Autodesk Fusion 360 part; units mm, degrees
(part 2 of 2)
sketch "Skizze6" plane through (0, 45, 0) normal (0, 1, 0) x (-1, 0, 0) in component "Board"
  circle A0 centre (45, 23.5) radius 1.5
  circle A1 centre (-94.5, -90.5) radius 1.5
  circle A2 centre (45, -90.5) radius 1.5
  circle A3 centre (-94.5, 23.5) radius 1.5
  line L0 (-104.5, -100.5) -> (55, -100.5)
  line L1 (55, -100.5) -> (55, 33.5)
  line L2 (55, 33.5) -> (-104.5, 33.5)
  line L3 (-104.5, 33.5) -> (-104.5, -100.5)
  circle A4 centre (-94.5, -90.5) radius 3
  circle A5 centre (45, -90.5) radius 3
  circle A6 centre (45, 23.5) radius 3
  circle A7 centre (-94.5, 23.5) radius 3
  dimension "d85" = 6
  dimension "d86" = 6
  dimension "d87" = 6
  dimension "d88" = 6
  constraint concentric A1 A4
  constraint concentric A2 A5
  constraint concentric A0 A6
  constraint concentric A3 A7
  measures "d85" diameter of A4
  measures "d86" diameter of A5
  measures "d87" diameter of A6
  measures "d88" diameter of A7
extrude "Extrusion12" cut sketch "Skizze6" against normal blind 3 contours A4 | A5 | A6 | A7 bodies 3 in component "Board"
sketch "Skizze7" plane through (104.5, 0, 0) normal (1, 0, 0) x (0, 0, -1) in component "Board"
  line L0 (100.5, -5) -> (100.5, 40)
  line L1 (100.5, 40) -> (-33.5, 40)
  line L2 (-33.5, 40) -> (-33.5, -5)
  line L3 (-33.5, -5) -> (100.5, -5)
  line L4 (41.5, 0) -> (25.5, 0)
  line L5 (25.5, 0) -> (41.5, 0)
  line L6 (60.5, 0) -> (51.5, 0)
  line L7 (47.25, 0) -> (60.5, 0)
  line L8 (25.5, 0) -> (60.5, 0) construction
  line L9 (60.5, 8) -> (25.5, 8) construction
  line L10 (25.5, 8) -> (25.5, 0) construction
  line L11 (25.5, 8) -> (73.5, 8) construction
  line L12 (73.5, 8) -> (73.5, 9.75) construction
  line L13 (73.5, 9.75) -> (25.5, 9.75) construction
  line L14 (25.5, 9.75) -> (25.5, 8) construction
  line L15 (25.5, 0) -> (41.5, 0) construction
  line L16 (41.5, 0) -> (41.5, 9.75) construction
  line L17 (41.5, 9.75) -> (25.5, 9.75) construction
  line L18 (25.5, 9.75) -> (25.5, 0) construction
  line L19 (60.5, 0) -> (51.5, 0) construction
  line L20 (51.5, 0) -> (51.5, 9.75) construction
  line L21 (51.5, 9.75) -> (60.5, 9.75) construction
  line L22 (25.5, 9.75) -> (42, 9.75)
  line L23 (42, 9.75) -> (42, 23.75)
  line L24 (42, 23.75) -> (25.5, 23.75)
  line L25 (25.5, 23.75) -> (25.5, 9.75)
  line L26 (51.5, 9.75) -> (73.5, 9.75)
  line L27 (73.5, 9.75) -> (73.5, 14.25)
  line L28 (73.5, 14.25) -> (51.5, 14.25)
  line L29 (51.5, 14.25) -> (51.5, 9.75)
  circle A0 centre (54, 12) radius 1.5
  circle A1 centre (71, 12) radius 1.5
  line L30 (57.5, 13.5) -> (67.5, 13.5)
  line L31 (67.5, 13.5) -> (67.5, 10.5)
  line L32 (67.5, 10.5) -> (57.5, 10.5)
  line L33 (57.5, 10.5) -> (57.5, 13.5)
  point P0 (41.5, 0)
  point P1 (25.5, 0)
  point P2 (60.5, 0)
  point P3 (51.5, 0)
  dimension "d91" = 8
  dimension "d92" = 1.75
  dimension "d93" = 14
  dimension "d103" = 22
  dimension "d104" = 17
  dimension "d107" = 2.5
  dimension "d119" = 2.25
  dimension "d120" = 2.25
  dimension "d121" = 2.5
  dimension "d122" = 2.5
  dimension "d125" = 3
  dimension "d126" = 10
  dimension "d127" = 0.75
  dimension "d128" = 0.75
  dimension "d175" = 16.5
  dimension "d176" = 3
  dimension "d177" = 3
  constraint horizontal L8
  constraint horizontal L9
  constraint vertical L10
  constraint coincident P1 L4.end
  constraint horizontal L11
  constraint vertical L12
  constraint horizontal L13
  constraint vertical L14
  constraint horizontal L15
  constraint vertical L16
  constraint horizontal L17
  constraint vertical L18
  constraint coincident L13 L16.end
  constraint horizontal L19
  constraint vertical L20
  constraint horizontal L21
  constraint coincident L13 L20.end
  constraint coincident P2 L6.start
  constraint horizontal L22
  constraint vertical L23
  constraint horizontal L24
  constraint vertical L25
  constraint horizontal L26
  constraint vertical L27
  constraint horizontal L28
  constraint vertical L29
  constraint horizontal L30
  constraint vertical L31
  constraint horizontal L32
  constraint vertical L33
  measures "d91" distance of P1 L9.end
  measures "d92" distance of L9.end L13.end
  measures "d93" distance of L13.end L24.end
  measures "d103" distance of L20.end L12.end
  measures "d104" horizontal distance of A0.centre A1.centre
  measures "d107" distance of L27 A1.centre
  measures "d119" distance of L13 A0.centre
  measures "d120" distance of L28 A0.centre
  measures "d121" distance of L29 A0.centre
  measures "d122" distance of L27 A1.centre
  measures "d125" distance of L30.start L32.end
  measures "d126" distance of L31.end L32.end
  measures "d127" distance of L13 L31.end
  measures "d128" distance of L28 L30.end
  measures "d175" distance of L23.end L24.end
  measures "d176" diameter of A0
  measures "d177" diameter of A1
extrude "Extrusion13" cut sketch "Skizze7" against normal up to surface (5 mm away) contours L22 L23 L24 L25 | A0 | A1 | L30 L31 L32 L33 bodies 2 in component "Board"
chamfer "Fase2" distance 3.5 angle 45 4 edges at (104.5, 16.75, -42) (104.5, 23.75, -33.75) (104.5, 9.75, -33.75) (104.5, 16.75, -25.5) tangent chain off on bodies 2 in component "Board"
chamfer "Fase3" distance 5 angle 45 8 edges at (-55, 17.5, 33.5) (104.5, 17.5, 33.5) (104.5, 17.5, -100.5) (-55, 17.5, -100.5) (-55, 42.5, 33.5) (104.5, 42.5, 33.5) (104.5, 42.5, -100.5) (-55, 42.5, -100.5) on bodies 2 3 in component "Board"
sketch "Skizze9" plane through (0, 45, 0) normal (0, 1, 0) x (-1, 0, 0) in component "Board"
  line L0 (50, -100.5) -> (55, -95.5)
  line L1 (55, -95.5) -> (55, 28.5)
  line L2 (55, 28.5) -> (50, 33.5)
  line L3 (50, 33.5) -> (-99.5, 33.5)
  line L4 (-99.5, 33.5) -> (-104.5, 28.5)
  line L5 (-104.5, 28.5) -> (-104.5, -95.5)
  line L6 (-104.5, -95.5) -> (-99.5, -100.5)
  line L7 (-99.5, -100.5) -> (50, -100.5)
  circle A0 centre (-94.5, -90.5) radius 3
  circle A1 centre (-94.5, 23.5) radius 3
  circle A2 centre (45, -90.5) radius 3
  circle A3 centre (45, 23.5) radius 3
  line L8 (43.8594, -20.5) -> (32.3594, -20.5)
  line L9 (32.3594, -20.5) -> (32.3594, -50.5)
  line L10 (32.3594, -50.5) -> (43.8594, -50.5)
  line L11 (43.8594, -50.5) -> (43.8594, -20.5)
  line L12 (-24.75, 33.5) -> (-24.75, -100.5)
  line L13 (-104.5, -33.5) -> (55, -33.5)
  line L14 (-24.75, -96.6299) -> (-24.75, 29.6299) construction
  line L15 (-24.75, 29.6299) -> (-24.8533, 29.6299) construction
  line L16 (-24.8533, 29.6299) -> (-24.8533, -96.6299) construction
  line L17 (-24.8533, -96.6299) -> (-24.75, -96.6299) construction
  line L18 (32.3594, -50.5) -> (43.8594, -20.5) construction
  line L19 (32.3594, -20.5) -> (43.8594, -50.5) construction
  line L20 (32.1094, -53) -> (44.1094, -53)
  line L21 (44.1094, -53) -> (44.1094, -14)
  line L22 (44.1094, -14) -> (32.1094, -14)
  line L23 (32.1094, -14) -> (32.1094, -53)
  line L24 (32.1094, -53) -> (44.1094, -14) construction
  line L25 (44.1094, -53) -> (32.1094, -14) construction
  dimension "d109" = 11.5
  dimension "d110" = 30
  dimension "d115" = 20
  dimension "d133" = 39
  dimension "d134" = 12
  dimension "d135" = 6.5
  dimension "d136" = 13
  text T0 "sACN Node" font "Arial" height 20 align centre middle in box 126.2599 x 0.1033 at (-24.75, -96.6299) x (0, 1) y (-1, 0) spacing 1 kerned
  constraint horizontal L8
  constraint vertical L9
  constraint horizontal L10
  constraint vertical L11
  constraint midpoint L3 L12.start
  constraint midpoint L7 L12.end
  constraint midpoint L5 L13.start
  constraint midpoint L1 L13.end
  constraint coincident L12
  constraint midpoint L12
  constraint horizontal L20
  constraint perpendicular L20 L21
  constraint parallel L20 L22
  constraint parallel L21 L23
  measures "d109" distance of L8.start L8.end
  measures "d110" distance of L8.start L10.end
  measures "d133" distance of L20.end L21.end
  measures "d134" distance of L21.end L22.end
  measures "d135" vertical distance of L8.end L22.end
  measures "d136" distance of L8 L13
extrude "Extrusion15" cut sketch "Skizze9" against normal blind 6 contours L8 L9 L11 L13 | L9 L10 L11 L13 bodies 3 in component "Board"
extrude "Extrusion16" cut sketch "Skizze9" against normal blind 2 text T0 bodies 3 in component "Board"
extrude "Extrusion17" cut sketch "Skizze7" against normal blind 3.6 contours L26 L27 L28 L29 bodies 2 in component "Board"
chamfer "Fase5" distance 3.6 angle 45 4 edges at (104.5, 14.25, -62.5) (104.5, 12, -51.5) (104.5, 9.75, -62.5) (104.5, 12, -73.5) on bodies 2 in component "Board"
combine "Kombinieren1" operation add target body 2 tool bodies 6 7 5 4 in component "Board"
sketch "Skizze5 (2)" plane through (0, 40.6077, 0) normal (0, -1, 0) x (1, 0, 0)
  line L0 (-44.0592, -20.4704) -> (-32.5592, -20.4704)
  line L1 (-32.5592, -20.4704) -> (-32.5592, -50.4704)
  line L2 (-32.5592, -50.4704) -> (-44.0592, -50.4704)
  line L3 (-44.0592, -50.4704) -> (-44.0592, -20.4704)
  circle A0 centre (-45.1999, 23.5296) radius 1.5
  circle A1 centre (94.3001, -90.4704) radius 1.5
  circle A2 centre (-45.1999, -90.4704) radius 1.5
  circle A3 centre (94.3001, 23.5296) radius 1.5
  line L4 (-55.1999, -95.4704) -> (-50.1999, -100.4704)
  line L5 (-50.1999, -100.4704) -> (99.3001, -100.4704)
  line L6 (99.3001, -100.4704) -> (104.3001, -95.4704)
  line L7 (104.3001, -95.4704) -> (104.3001, 28.5296)
  line L8 (104.3001, 28.5296) -> (99.3001, 33.5296)
  line L9 (99.3001, 33.5296) -> (-50.1999, 33.5296)
  line L10 (-50.1999, 33.5296) -> (-55.1999, 28.5296)
  line L11 (-55.1999, 28.5296) -> (-55.1999, -95.4704)
  line L12 (-32.5592, -50.4704) -> (-44.0592, -50.4704) construction
  line L13 (-44.0592, -50.4704) -> (-44.0592, -20.4704) construction
  line L14 (-44.0592, -20.4704) -> (-32.5592, -20.4704) construction
  line L15 (-32.5592, -20.4704) -> (-32.5592, -50.4704) construction
  line L16 (-32.0592, -57.2204) -> (-44.5592, -57.2204)
  line L17 (-44.5592, -57.2204) -> (-44.5592, -18.7204)
  line L18 (-44.5592, -18.7204) -> (-32.0592, -18.7204)
  line L19 (-32.0592, -18.7204) -> (-32.0592, -57.2204)
  line L20 (-32.5592, -50.4704) -> (-44.0592, -50.4704) construction
  line L21 (-44.0592, -50.4704) -> (-44.0592, -20.4704) construction
  line L22 (-44.0592, -20.4704) -> (-32.5592, -20.4704) construction
  line L23 (-32.5592, -20.4704) -> (-32.5592, -50.4704) construction
  dimension "d155" = 11.5
  dimension "d156" = 30
  dimension "d157" = 12.5
  dimension "d158" = 38.5
  dimension "d159" = 1.75
  dimension "d160" = 0.5
  constraint horizontal L12
  constraint vertical L13
  constraint horizontal L14
  constraint vertical L15
  constraint coincident L0.start L3.end
  constraint coincident L1.end L2.start
  constraint horizontal L16
  constraint vertical L17
  constraint horizontal L18
  constraint vertical L19
  constraint horizontal L20
  constraint vertical L21
  constraint horizontal L22
  constraint vertical L23
  measures "d155" distance of L1.end L2.end
  measures "d156" distance of L0.end L1.end
  measures "d157" distance of L16.start L16.end
  measures "d158" distance of L16.start L18.end
  measures "d159" distance of L14 L18
  measures "d160" distance of L19 L23
sketch "Skizze6 (2)" plane through (99.3001, 0, 0) normal (-1, 0, 0) x (0, 0, 1)
  line L0 (-42.2204, 5.6077) -> (-42.2204, 40.6077)
  line L1 (-42.2204, 40.6077) -> (-85.4704, 40.6077)
  line L2 (-85.4704, 40.6077) -> (-85.4704, 30.6077)
  line L3 (-85.4704, 30.6077) -> (-95.4704, 20.6077)
  line L4 (-95.4704, 20.6077) -> (-95.4704, 0.6077)
  line L5 (-57.4704, 14.1077) -> (-57.4704, 11.1077)
  line L6 (-57.4704, 11.1077) -> (-67.4704, 11.1077)
  line L7 (-67.4704, 11.1077) -> (-67.4704, 14.1077)
  line L8 (-67.4704, 14.1077) -> (-57.4704, 14.1077)
  circle A0 centre (-70.9704, 12.6077) radius 1.5
  circle A1 centre (-53.9704, 12.6077) radius 1.5
  line L9 (-47.2204, 5.6077) -> (-42.2204, 5.6077)
  line L10 (-95.4704, 0.6077) -> (-47.2204, 0.6077)
  line L11 (-47.2204, 0.6077) -> (-47.2204, 5.6077)
sketch "Skizze9 (2)" plane through (99.3001, 0, 0) normal (-1, 0, 0) x (0, 0, 1)
  line L0 (-49.9704, 18.6077) -> (-74.9704, 18.6077)
  line L1 (-74.9704, 18.6077) -> (-74.9704, 6.6077)
  line L2 (-74.9704, 6.6077) -> (-49.9704, 6.6077)
  line L3 (-49.9704, 6.6077) -> (-49.9704, 18.6077)
  line L4 (-67.4704, 14.1077) -> (-57.4704, 14.1077)
  line L5 (-57.4704, 11.1077) -> (-67.4704, 11.1077)
  line L6 (-67.4704, 11.1077) -> (-67.4704, 14.1077)
  line L7 (-57.4704, 14.1077) -> (-57.4704, 11.1077)
  dimension "d167" = 25
  dimension "d168" = 12
  dimension "d169" = 4.5
  dimension "d170" = 4.5
  dimension "d171" = 7.5
  dimension "d172" = 7.5
  constraint horizontal L0
  constraint vertical L1
  constraint horizontal L2
  constraint vertical L3
  measures "d167" distance of L0.start L0.end
  measures "d168" distance of L0.start L2.end
  measures "d169" distance of L0 L4
  measures "d170" distance of L2 L5
  measures "d171" distance of L1 L6
  measures "d172" distance of L3 L7
extrude "Extrusion22" cut sketch "Skizze9 (2)" against normal blind 1 sketch seen with x (1, 0, 0) y (0, 1, 0) z (0, 0, 1) at (0.1999, -0.6077, -0.0296) bodies 2 in component "Board"
extrude "Extrusion21" cut sketch "Skizze5 (2)" against normal blind 4.6 contours L16 L17 L18 L19 sketch seen with x (1, 0, 0) y (0, 1, 0) z (0, 0, 1) at (0.1999, -0.6077, -0.0296) bodies 3 in component "Board"
extrude "Extrusion1'" add sketch "Skizze1" along normal blind 7 separate body contours L34 L36 L72 L78 L99 L103 L120 L125 | L41 L45 L55 L67 L88 L91 L105 L126 | L153 L156 L157 L171 L182 L185 L193 L197 | L166 L175 L180 L181 L187 L195 L198 L199 | L249 L253 L254 L269 L280 L284 L293 L297 | L264 L273 L278 L279 L286 L295 L298 L299 | L349 L353 L354 L369 L380 L384 L393 L397 | L364 L373 L378 L379 L386 L395 L398 L399 in plane through (0, 4.3947, 0) normal (0, 1, 0) sketch seen with x (1, 0, 0) y (0, 1, 0) z (0, 0, 1) at (-0.1999, 0.6077, 0.0296) makes body 8 at (-2.5127, 9.6691, -8.9481) makes body 9 at (-2.5127, 9.6691, -69.9481) makes body 10 at (1.4869, 7.3358, -77.9816) makes body 11 at (-2.5127, 9.6691, -14.9816) makes body 12 at (-2.5127, 9.6691, 15.5184) makes body 13 at (1.4873, 7.3358, -47.4816) makes body 14 at (-2.5127, 9.6691, 21.5519) makes body 15 at (-2.5127, 9.6691, -41.4481)
sketch "Skizze10" plane through (0, 0, 0) normal (0, 1, 0) x (1, 0, 0)
component "Board" placed x (1, 0, 0) y (0, 1, 0) z (0, 0, 1) at (-0.1999, 0.6077, 0.0296)
equation "d116 = 'sACN Node'"
named bodies: "BasePlate", "MainShell", "Lid"
